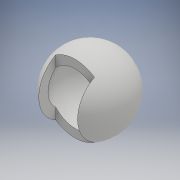
# Autodesk Inventor part: Деталь_4
Saved by Autodesk Inventor 2019.3 (Build 233278000, 278)
## iProperties
Created: 2020-03-16
Part Number: Деталь_4
Material: Типовые
Document SubType Name: Modeling
Designer: Diana
Density: 1 g/cm^3
Appearance: По умолчанию
Author: Diana
Autodesk Inventor part; units mm, degrees
ref_plane "YZ Plane" through (0, 0, 0) normal (1, 0, 0) x (0, 1, 0)
ref_plane "XZ Plane" through (0, 0, 0) normal (0, 1, 0) x (-1, 0, 0)
ref_plane "XY Plane" through (0, 0, 0) normal (0, 0, 1) x (1, 0, 0)
sketch "Эскиз1" plane through (0, 0, 0) normal (0, 0, 1) x (1, 0, 0)
  arc A0 (0, -25) -> (0, 25) centre (0, 0) ccw
  arc A1 (0, -20) -> (0, 20) centre (0, 0) ccw
  line L0 (0, 25) -> (0, 20)
  line L1 (0, -20) -> (0, -25)
  line L2 (0, -35) -> (0, 35) projected
  dimension "d0" = 20
  dimension "d1" = 25
  constraints: 4 end point, 4 point on circle, 4 vertical alignment, 3 coincident, 2 centre point, 2 vertical, 1 other
  measures "d0" radius of A1
  measures "d1" radius of A0
revolve "Вращение1" add sketch "Эскиз1" angle 360 about axis through (0, -10, 0) along (0, 1, 0) contours L1 A1 L0 A0
sketch "Эскиз2" plane through (0, 0, 0) normal (0, 0, 1) x (1, 0, 0)
  circle A0 centre (0, 0) radius 13
  dimension "d3" = 26
  constraints: 1 centre point, 1 coincident, 1 other
  measures "d3" diameter of A0
extrude "Выдавливание1" cut sketch "Эскиз2" against normal through all
sketch "Эскиз3" plane through (0, 0, 0) normal (0, 1, 0) x (-1, 0, 0)
  arc A0 (13, -21.3542) -> (-13, -21.3542) centre (0, 0) ccw projected
  line L0 (13, 10) -> (-13, 10)
  line L1 (-13, 10) -> (-13, 25)
  line L2 (-13, 25) -> (13, 25)
  line L3 (13, 25) -> (13, 10)
  dimension "d6" = 10
  dimension "d7" = 26
  dimension "d9" = 13
  constraints: 8 end point, 2 parallel, 1 horizontal, 1 perpendicular, 1 tangent
  measures "d6" distance from line of L0 point (0, 0)
  measures "d7" distance of L1.end L2.end
  measures "d9" distance from line of L1 point (0, 0)
extrude "Выдавливание2" cut sketch "Эскиз3" along normal through all both and the other way through all
